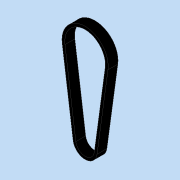
# Autodesk Inventor part: Pas zębaty 10 T5-275
Saved by Autodesk Inventor 2018 (Build 220112000, 112)
## iProperties
Created: 2019-02-09
Part Number: Pas zębaty 10 T5-275
Material: Ogólny
Document SubType Name: Modeling
Designer: Dawid
Density: 1 g/cm^3
Appearance: Anodowana - czarna
Author: Dawid
Autodesk Inventor part; units mm, degrees
ref_plane "YZ Plane" through (0, 0, 0) normal (1, 0, 0) x (0, 1, 0)
ref_plane "XZ Plane" through (0, 0, 0) normal (0, 1, 0) x (-1, 0, 0)
ref_plane "XY Plane" through (0, 0, 0) normal (0, 0, 1) x (1, 0, 0)
sketch "Szkic1" plane through (0, 0, 0) normal (0, 1, 0) x (-1, 0, 0)
  line L0 (15.3323, 42.2692) -> (20.2794, 78.2084)
  line L1 (-14.2554, 34.4465) -> (-9.3368, -1.2852)
  line L2 (-14.2554, 34.4465) -> (-20.2794, 78.2084)
  arc A0 (20.2794, 78.2084) -> (-20.2794, 78.2084) centre (0, 81) ccw
  arc A1 (-12.1108, -1.6671) -> (12.1108, -1.6671) centre (0, 0) ccw
  arc A2 (-12.1108, -1.6671) -> (12.1108, -1.6671) centre (0, 0) ccw
  line L3 (23.1567, 77.8124) -> (12.1108, -1.6671)
  line L4 (-12.1108, -1.6671) -> (-23.1566, 77.8124)
  arc A3 (-9.3368, -1.2852) -> (9.3368, -1.2852) centre (0, 0) ccw
  arc A4 (23.1483, 77.7522) -> (-23.1483, 77.7523) centre (0, 81) ccw
  line L5 (15.3323, 42.2692) -> (9.3368, -1.2852)
  point P0 (0, 0)
  constraints: 12 end point, 12 point on circle, 5 centre point, 2 coincident, 2 point on line, 4 other
extrude "Wyciągnięcie proste1" add sketch "Szkic1" along normal blind 10
